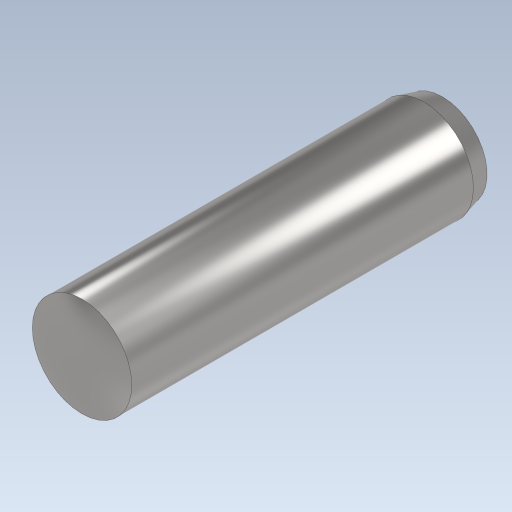
# Autodesk Inventor part: _SPA-SUS-D1.6-6
Saved by Autodesk Inventor 2024 (Build 280153000, 153)
## iProperties
Created: 2023-09-03
Part Number: _SPA-SUS-D1.6-6
Material: ステンレス鋼
Document SubType Name: Modeling
Designer: michi
Density: 8 g/cm^3
Appearance: 半つや出し
Author: michi
Autodesk Inventor part; units mm, degrees
ref_plane "YZ Plane" through (0, 0, 0) normal (1, 0, 0) x (0, 1, 0)
ref_plane "XZ Plane" through (0, 0, 0) normal (0, 1, 0) x (-1, 0, 0)
ref_plane "XY Plane" through (0, 0, 0) normal (0, 0, 1) x (1, 0, 0)
sketch "スケッチ1" plane through (0, 0, 0) normal (1, 0, 0) x (0, 1, 0)
  line L0 (0, 3) -> (0.8, 3)
  line L1 (0.8, 3) -> (0.8, -3)
  line L2 (0.8, -3) -> (0, -3)
  line L3 (0, -3) -> (0, 3)
  line L4 (0.8, -2.7) -> (0.7196, -3)
  arc A0 (0.8, 2.8) -> (0, 3) centre (0, 1.3) ccw
  point P0 (0, 0)
  point P1 (0, 0)
  dimension "d0" = 1.6
  dimension "d1" = 6
  dimension "d3" = 0.2
  dimension "d4" = 0.3
  dimension "d5" = 15
  constraints: 10 end point, 3 point on line, 2 parallel, 2 point on circle, 1 centre point, 1 coincident, 1 horizontal, 1 midpoint, 1 perpendicular, 1 tangent
  measures "d0" diameter of L1 L3
  measures "d1" distance of L0.end L1.end
  measures "d3" distance from line of L0 A0.start
  measures "d4" vertical distance of L4.start L4.end
  measures "d5" angle of L1 L4
revolve "回転1" add sketch "スケッチ1" angle 360 about axis through (0, 0, -3) along (0, 0, 1) contours A0 L1 L4 L2 L3
